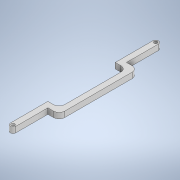
# Autodesk Inventor part: Балка рулевого управления
Saved by Autodesk Inventor 2020 (Build 240168000, 168)
## iProperties
Created: 2021-03-21
Part Number: Балка рулевого управления
Material: Типовые
Document SubType Name: Modeling
Designer: Антон
Density: 1 g/cm^3
Appearance: По умолчанию
Author: Антон
Autodesk Inventor part; units mm, degrees
ref_plane "YZ Plane" through (0, 0, 0) normal (1, 0, 0) x (0, 1, 0)
ref_plane "XZ Plane" through (0, 0, 0) normal (0, 1, 0) x (-1, 0, 0)
ref_plane "XY Plane" through (0, 0, 0) normal (0, 0, 1) x (1, 0, 0)
sketch "Эскиз1" plane through (0, 0, 0) normal (0, 1, 0) x (-1, 0, 0)
  line L0 (0, 0) -> (5, 0)
  line L1 (5, 0) -> (5, -66)
  line L2 (5, -66) -> (0, -66)
  line L3 (0, -66) -> (0, 0)
  line L4 (2.5, 0) -> (2.5, -2.5)
  circle A0 centre (2.5, -2.5) radius 1.5
  line L5 (0, -66) -> (-10, -66)
  line L6 (-10, -66) -> (-10, -31)
  line L7 (-10, -31) -> (0, -31)
  line L8 (0, -31) -> (0, -66)
  line L9 (5, -66) -> (0, -66)
  line L10 (5, -66) -> (-5, -66)
  line L11 (-5, -66) -> (-5, -36)
  line L12 (-5, -36) -> (5, -36)
  line L13 (5, -36) -> (5, -66)
  point P0 (0, -31)
  point P1 (0, -36)
  point P2 (5, -36)
  dimension "d0" = 5
  dimension "d1" = 66
  dimension "d4" = 2.5
  dimension "d5" = 3
  dimension "d7" = 10
  dimension "d8" = 35
  dimension "d11" = 10
  dimension "d12" = 30
  constraints: 28 end point, 6 parallel, 4 horizontal, 3 perpendicular, 1 centre point, 1 coincident, 1 midpoint, 1 vertical
  measures "d0" distance of L1.end L2.end
  measures "d1" distance of L0.end L1.end
  measures "d4" distance of L4.start L4.end
  measures "d5" diameter of A0
  measures "d7" distance of L6.end L7.end
  measures "d8" distance of L5.end L6.end
  measures "d11" distance of L11.end L12.end
  measures "d12" distance of L10.end L11.end
extrude "Выдавливание1" add sketch "Эскиз1" along normal blind 5 contours L0 L1 L12 L3 | L3 L12 L11 L5 L6 L7
fillet "Сопряжение1" radius 2.5 2 edges at (0, 2.5, 0) (-5, 2.5, 0)
fillet "Сопряжение2" radius 5 2 edges at (10, 2.5, -31) (5, 2.5, -36)
mirror "Зеркальное отражение2" about plane through (10, 0, -66) normal (0, 0, -1)
equation "\"d11\" = d7"
equation "\"d12\" = d8 - d0"
